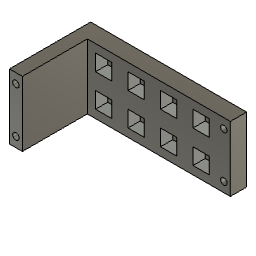
cementform_rect_80x40_plateA (Autodesk Fusion 360 design; units mm, degrees)
Autodesk Fusion 360 part; units mm, degrees
sketch "baseplate" plane through (0, 0, 0) normal (0, 1, 0) x (1, 0, 0)
  line L0 (0, 0) -> (80, 0)
  line L1 (80, 0) -> (80, -40)
  line L2 (80, -40) -> (0, -40)
  line L3 (0, -40) -> (0, 0)
  dimension "d1" = 40
  dimension "d2" = 80
  constraint horizontal L0
  constraint vertical L1
  constraint horizontal L2
  constraint vertical L3
  constraint coincident L0.start L3.end
  measures "d1" distance of L0.start L2.end
  measures "d2" distance of L0.start L0.end
extrude "Extrude1" add sketch "baseplate" along normal blind 10
sketch "outside_pryamid" plane through (0, 0, 0) normal (0, 1, 0) x (1, 0, 0)
  line L0 (5, -35) -> (15, -35)
  line L1 (15, -35) -> (15, -25)
  line L2 (15, -25) -> (5, -25)
  line L3 (5, -25) -> (5, -35)
  line L4 (25, -35) -> (35, -35)
  line L5 (35, -35) -> (35, -25)
  line L6 (35, -25) -> (25, -25)
  line L7 (25, -25) -> (25, -35)
  line L8 (45, -35) -> (55, -35)
  line L9 (55, -35) -> (55, -25)
  line L10 (55, -25) -> (45, -25)
  line L11 (45, -25) -> (45, -35)
  line L12 (65, -35) -> (75, -35)
  line L13 (75, -35) -> (75, -25)
  line L14 (75, -25) -> (65, -25)
  line L15 (65, -25) -> (65, -35)
  line L16 (25, -15) -> (35, -15)
  line L17 (35, -15) -> (35, -5)
  line L18 (35, -5) -> (25, -5)
  line L19 (25, -5) -> (25, -15)
  line L20 (5, -15) -> (15, -15)
  line L21 (15, -15) -> (15, -5)
  line L22 (15, -5) -> (5, -5)
  line L23 (5, -5) -> (5, -15)
  line L24 (45, -15) -> (55, -15)
  line L25 (55, -15) -> (55, -5)
  line L26 (55, -5) -> (45, -5)
  line L27 (45, -5) -> (45, -15)
  line L28 (65, -15) -> (75, -15)
  line L29 (75, -15) -> (75, -5)
  line L30 (75, -5) -> (65, -5)
  line L31 (65, -5) -> (65, -15)
  dimension "d5" = 10
  dimension "d6" = 10
  constraint horizontal L0
  constraint vertical L1
  constraint horizontal L2
  constraint vertical L3
  constraint horizontal L4
  constraint vertical L5
  constraint horizontal L6
  constraint vertical L7
  constraint horizontal L8
  constraint vertical L9
  constraint horizontal L10
  constraint vertical L11
  constraint horizontal L12
  constraint vertical L13
  constraint horizontal L14
  constraint vertical L15
  constraint horizontal L16
  constraint vertical L17
  constraint horizontal L18
  constraint vertical L19
  constraint horizontal L20
  constraint vertical L21
  constraint horizontal L22
  constraint vertical L23
  constraint horizontal L24
  constraint vertical L25
  constraint horizontal L26
  constraint vertical L27
  constraint horizontal L28
  constraint vertical L29
  constraint horizontal L30
  constraint vertical L31
  measures "d5" distance of L20.start L20.end
  measures "d6" distance of L20.start L22.end
ref_plane "WorkPlane1" through (0, 5, 0) normal (0, 1, 0) x (0, 0, 1)
sketch "inside_pryamid" plane through (0, 5, 0) normal (0, 1, 0) x (1, 0, 0)
  line L0 (7.5, -10) -> (7.5, -12.5)
  line L1 (7.5, -12.5) -> (12.5, -12.5)
  line L2 (12.5, -12.5) -> (12.5, -7.5)
  line L3 (12.5, -7.5) -> (7.5, -7.5)
  line L4 (7.5, -7.5) -> (7.5, -10)
  line L5 (32.5, -7.5) -> (27.5, -7.5)
  line L6 (27.5, -10) -> (27.5, -12.5)
  line L7 (32.5, -12.5) -> (32.5, -7.5)
  line L8 (27.5, -7.5) -> (27.5, -10)
  line L9 (27.5, -12.5) -> (32.5, -12.5)
  line L10 (47.5, -7.5) -> (47.5, -10)
  line L11 (47.5, -12.5) -> (52.5, -12.5)
  line L12 (52.5, -7.5) -> (47.5, -7.5)
  line L13 (47.5, -10) -> (47.5, -12.5)
  line L14 (52.5, -12.5) -> (52.5, -7.5)
  line L15 (67.5, -10) -> (67.5, -12.5)
  line L16 (67.5, -12.5) -> (72.5, -12.5)
  line L17 (67.5, -7.5) -> (67.5, -10)
  line L18 (72.5, -12.5) -> (72.5, -7.5)
  line L19 (72.5, -7.5) -> (67.5, -7.5)
  line L20 (67.5, -10) -> (67.5, -12.5)
  line L21 (7.5, -7.5) -> (7.5, -10)
  line L22 (12.5, -7.5) -> (7.5, -7.5)
  line L23 (7.5, -10) -> (7.5, -12.5)
  line L24 (67.5, -12.5) -> (72.5, -12.5)
  line L25 (27.5, -10) -> (27.5, -12.5)
  line L26 (27.5, -12.5) -> (32.5, -12.5)
  line L27 (7.5, -12.5) -> (12.5, -12.5)
  line L28 (32.5, -12.5) -> (32.5, -7.5)
  line L29 (72.5, -12.5) -> (72.5, -7.5)
  line L30 (47.5, -7.5) -> (47.5, -10)
  line L31 (52.5, -12.5) -> (52.5, -7.5)
  line L32 (72.5, -7.5) -> (67.5, -7.5)
  line L33 (47.5, -10) -> (47.5, -12.5)
  line L34 (52.5, -7.5) -> (47.5, -7.5)
  line L35 (67.5, -7.5) -> (67.5, -10)
  line L36 (47.5, -12.5) -> (52.5, -12.5)
  line L37 (32.5, -7.5) -> (27.5, -7.5)
  line L38 (27.5, -7.5) -> (27.5, -10)
  line L39 (12.5, -12.5) -> (12.5, -7.5)
  line L40 (72.5, -32.5) -> (72.5, -27.5)
  line L41 (12.5, -32.5) -> (12.5, -27.5)
  line L42 (72.5, -27.5) -> (67.5, -27.5)
  line L43 (7.5, -30) -> (7.5, -32.5)
  line L44 (67.5, -30) -> (67.5, -32.5)
  line L45 (72.5, -27.5) -> (67.5, -27.5)
  line L46 (67.5, -27.5) -> (67.5, -30)
  line L47 (47.5, -30) -> (47.5, -32.5)
  line L48 (12.5, -27.5) -> (7.5, -27.5)
  line L49 (67.5, -27.5) -> (67.5, -30)
  line L50 (67.5, -30) -> (67.5, -32.5)
  line L51 (7.5, -32.5) -> (12.5, -32.5)
  line L52 (67.5, -32.5) -> (72.5, -32.5)
  line L53 (72.5, -32.5) -> (72.5, -27.5)
  line L54 (7.5, -30) -> (7.5, -32.5)
  line L55 (47.5, -32.5) -> (52.5, -32.5)
  line L56 (47.5, -32.5) -> (52.5, -32.5)
  line L57 (67.5, -32.5) -> (72.5, -32.5)
  line L58 (52.5, -32.5) -> (52.5, -27.5)
  line L59 (7.5, -32.5) -> (12.5, -32.5)
  line L60 (52.5, -27.5) -> (47.5, -27.5)
  line L61 (52.5, -27.5) -> (47.5, -27.5)
  line L62 (47.5, -30) -> (47.5, -32.5)
  line L63 (7.5, -27.5) -> (7.5, -30)
  line L64 (27.5, -30) -> (27.5, -32.5)
  line L65 (32.5, -27.5) -> (27.5, -27.5)
  line L66 (27.5, -32.5) -> (32.5, -32.5)
  line L67 (52.5, -32.5) -> (52.5, -27.5)
  line L68 (27.5, -27.5) -> (27.5, -30)
  line L69 (32.5, -32.5) -> (32.5, -27.5)
  line L70 (27.5, -32.5) -> (32.5, -32.5)
  line L71 (27.5, -30) -> (27.5, -32.5)
  line L72 (12.5, -27.5) -> (7.5, -27.5)
  line L73 (7.5, -27.5) -> (7.5, -30)
  line L74 (47.5, -27.5) -> (47.5, -30)
  line L75 (12.5, -32.5) -> (12.5, -27.5)
  line L76 (47.5, -27.5) -> (47.5, -30)
  line L77 (32.5, -32.5) -> (32.5, -27.5)
  line L78 (32.5, -27.5) -> (27.5, -27.5)
  line L79 (27.5, -27.5) -> (27.5, -30)
  constraint perpendicular L0 L1
  constraint perpendicular L1 L2
  constraint perpendicular L2 L3
  constraint perpendicular L6 L9
  constraint perpendicular L7 L9
  constraint perpendicular L5 L7
  constraint perpendicular L11 L13
  constraint perpendicular L11 L14
  constraint perpendicular L12 L14
  constraint perpendicular L15 L16
  constraint perpendicular L16 L18
  constraint perpendicular L18 L19
  constraint perpendicular L23 L27
  constraint perpendicular L27 L39
  constraint perpendicular L22 L39
  constraint perpendicular L25 L26
  constraint perpendicular L26 L28
  constraint perpendicular L28 L37
  constraint perpendicular L33 L36
  constraint perpendicular L31 L36
  constraint perpendicular L31 L34
  constraint perpendicular L20 L24
  constraint perpendicular L24 L29
  constraint perpendicular L29 L32
  constraint perpendicular L54 L59
  constraint perpendicular L59 L75
  constraint perpendicular L72 L75
  constraint perpendicular L64 L70
  constraint perpendicular L69 L70
  constraint perpendicular L69 L78
  constraint perpendicular L47 L55
  constraint perpendicular L55 L67
  constraint perpendicular L61 L67
  constraint perpendicular L50 L57
  constraint perpendicular L53 L57
  constraint perpendicular L42 L53
  constraint perpendicular L43 L51
  constraint perpendicular L41 L51
  constraint perpendicular L41 L48
  constraint perpendicular L66 L71
  constraint perpendicular L66 L77
  constraint perpendicular L65 L77
  constraint perpendicular L56 L62
  constraint perpendicular L56 L58
  constraint perpendicular L58 L60
  constraint perpendicular L44 L52
  constraint perpendicular L40 L52
  constraint perpendicular L40 L45
loft "Loft1" cut profiles "outside_pryamid", "inside_pryamid" section 1 contours L0 L1 L2 L3 section 2 contours L41 L43 L48 L51 L54 L59 L63 L72 L73 L75
loft "Loft2" cut profiles "outside_pryamid", "inside_pryamid" section 1 contours L4 L5 L6 L7 section 2 contours L64 L65 L66 L68 L69 L70 L71 L77 L78 L79
loft "Loft3" cut profiles "outside_pryamid", "inside_pryamid" section 1 contours L8 L9 L10 L11 section 2 contours L47 L55 L56 L58 L60 L61 L62 L67 L74 L76
loft "Loft4" cut profiles "inside_pryamid", "outside_pryamid" section 1 contours L40 L42 L44 L45 L46 L49 L50 L52 L53 L57 section 2 contours L12 L13 L14 L15
loft "Loft5" cut profiles "inside_pryamid", "outside_pryamid" section 1 contours L0 L1 L2 L3 L4 L21 L22 L23 L27 L39 section 2 contours L20 L21 L22 L23
loft "Loft6" cut profiles "inside_pryamid", "outside_pryamid" section 1 contours L5 L6 L7 L8 L9 L25 L26 L28 L37 L38 section 2 contours L16 L17 L18 L19
loft "Loft7" cut profiles "inside_pryamid", "outside_pryamid" section 1 contours L10 L11 L12 L13 L14 L30 L31 L33 L34 L36 section 2 contours L24 L25 L26 L27
loft "Loft8" cut profiles "inside_pryamid", "outside_pryamid" section 1 contours L15 L16 L17 L18 L19 L20 L24 L29 L32 L35 section 2 contours L28 L29 L30 L31
sketch "sidewall" plane through (0, 0, 0) normal (0, 1, 0) x (1, 0, 0)
  line L0 (0, 0) -> (-8, 0)
  line L1 (-8, 0) -> (-8, -40)
  line L2 (-8, -40) -> (0, -40)
  line L3 (0, -40) -> (0, 0)
  dimension "d12" = 8
  constraint horizontal L0
  constraint vertical L1
  constraint horizontal L2
  constraint vertical L3
  constraint coincident L0.start L3.end
  measures "d12" distance of L1.end L2.end
extrude "Extrude2" add sketch "sidewall" along normal blind -40 and the other way blind -10
sketch "sidemount" plane through (0, 0, 0) normal (0, 1, 0) x (1, 0, 0)
  line L0 (80, 0) -> (88, 0)
  line L1 (88, 0) -> (88, -40)
  line L2 (88, -40) -> (80, -40)
  line L3 (80, -40) -> (80, 0)
  constraint horizontal L0
  constraint vertical L1
  constraint horizontal L2
  constraint vertical L3
extrude "Extrude3" add sketch "sidemount" along normal blind 10
sketch "Sketch6" plane through (0, 0, 0) normal (0, 1, 0) x (1, 0, 0)
  circle A0 centre (-4, -34) radius 2
  circle A1 centre (-4, -6) radius 2
  circle A2 centre (-4, -34) radius 3.4
  circle A3 centre (-4, -6) radius 3.4
  line L0 (88, 0) -> (84, 0)
  line L1 (84, 0) -> (84, -6)
  line L2 (84, -6) -> (88, -6)
  line L3 (88, -6) -> (88, 0)
  circle A4 centre (84, -34) radius 2
  circle A5 centre (84, -6) radius 2
  dimension "d19" = 4
  dimension "d20" = 4
  dimension "d21" = 6.8
  dimension "d22" = 6.8
  dimension "d25" = 4
  dimension "d26" = 6
  dimension "d27" = 4
  dimension "d28" = 4
  constraint concentric A0 A2
  constraint horizontal L0
  constraint vertical L1
  constraint horizontal L2
  constraint vertical L3
  constraint coincident L1.end L2.start
  measures "d19" diameter of A0
  measures "d20" diameter of A1
  measures "d21" diameter of A2
  measures "d22" diameter of A3
  measures "d25" distance of L0.start L0.end
  measures "d26" distance of L0.start L2.end
  measures "d27" diameter of A4
  measures "d28" diameter of A5
extrude "Extrude4" cut sketch "Sketch6" against normal blind 50 contours A0 | A1
extrude "Extrude5" cut sketch "Sketch6" along normal blind 40 contours L1 L2 A5 | L1 L2 A5 | A4
extrude "Extrude6" cut sketch "Sketch6" along normal through all and the other way blind 44 contours A0 | A1
extrude "Extrude7" cut sketch "Sketch6" along normal blind 10 and the other way blind -4 contours A2 | A3
